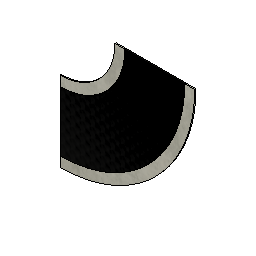
_End Turn - Ruby.f740c628-e54e-4ed0-8fb3-9d39286718e5 (Autodesk Fusion 360 design; units mm, degrees)
Autodesk Fusion 360 part; units mm, degrees
sketch "Sketch1" plane through (0, 0, 0) normal (0, 0, 1) x (1, 0, 0)
sketch "Sketch2" plane through (0, 0, 0) normal (0, 1, 0) x (1, 0, 0)
  circle A0 centre (-101.6, -254) radius 660.4
  circle A1 centre (-101.6, -254) radius 1270
  line L0 (-101.6, -254) -> (-101.6, -1524)
  line L1 (-101.6, -254) -> (1168.4, -254)
  line L2 (-101.6, -254) -> (-101.6, 1016)
  dimension "d1" = 1320.8
  dimension "d2" = 609.6
  constraint coincident A0.centre A1.centre
  constraint coincident A1 L0.end
  constraint vertical L0
  constraint coincident A1 L1.end
  constraint perpendicular L0 L1
  constraint coincident A1 L2.end
  constraint perpendicular L1 L2
  measures "d1" diameter of A0
extrude "Extrude1" add sketch "Sketch2" against normal blind 12.7 contours A0 A1 L1 L2 makes body 1
sketch "Sketch3" plane through (0, -12.7, 0) normal (0, -1, 0) x (1, 0, 0)
  arc A0 (-101.6, -1016) -> (1168.4, 254) centre (-101.6, 254) ccw
  line L0 (1168.4, 254) -> (558.8, 254)
  arc A1 (-101.6, -406.4) -> (558.8, 254) centre (-101.6, 254) ccw
  line L1 (-101.6, -406.4) -> (-101.6, -1016)
  line L2 (1266.2319, 355.6) -> (447.886, 355.6)
  arc A2 (-203.2, -295.486) -> (447.886, 355.6) centre (-101.6, 254) ccw
  line L3 (-203.2, -295.486) -> (-203.2, -1113.8319)
  arc A3 (-203.2, -1113.8319) -> (1266.2319, 355.6) centre (-101.6, 254) ccw
  line L4 (-101.6, -1016) -> (-101.6, -1117.6)
  line L5 (-101.6, -406.4) -> (-101.6, -304.8)
  line L6 (558.8, 254) -> (457.2, 254)
  line L7 (1168.4, 254) -> (1270, 254)
  dimension "d5" = -101.6
  constraint coincident A0.start L1.end
  constraint coincident A3 L4.end
  constraint parallel L1 L4
  constraint coincident A1.start L1.start
  constraint coincident A2 L5.end
  constraint parallel L1 L5
  constraint coincident L0.end A1.end
  constraint coincident A2 L6.end
  constraint perpendicular L5 L6
  constraint coincident A0.end L0.start
  constraint coincident A3 L7.end
  constraint parallel L0 L7
extrude "Extrude1'" add sketch "Sketch3" against normal blind 12.7 separate body contours A0 A3 L4 L7 | A1 A2 L5 L6 makes body 2 at (-70.2718, -12.7, -370.2927) makes body 3 at (1195.8119, -12.7, -59.1413) in component "Turn"
copy_body "CutPasteBodies1" bodies 1 removing the originals makes body 4 in component "Turn"
component "Turn" placed x (1, 0, 0) y (0, 1, 0) z (0, 0, 1) at (0, 0, 0)
